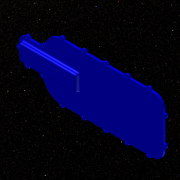
# Autodesk Inventor part: oilcaselid
Saved by Autodesk Inventor 2012 (Build 160160000, 160)
## iProperties
Created: 2012-11-14
Part Number: oilcaselid
Material: Default
Document SubType Name: Modeling
Designer: SONY
Density: 1 g/cm^3
Author: SONY
Autodesk Inventor part; units mm, degrees
ref_plane "YZ Plane" through (0, 0, 0) normal (1, 0, 0) x (0, 1, 0)
ref_plane "XZ Plane" through (0, 0, 0) normal (0, 1, 0) x (-1, 0, 0)
sketch "Sketch1" plane through (0, 0, 0) normal (0, 0, 1) x (1, 0, 0)
  circle A0 centre (150.6134, -24.6977) radius 1.778 projected
  circle A1 centre (150.6134, 24.5422) radius 1.778 projected
  circle A2 centre (122.2034, -53.1077) radius 1.778 projected
  circle A3 centre (122.2034, 52.9522) radius 1.778 projected
  circle A4 centre (-75.7202, -23.3991) radius 1.778 projected
  circle A5 centre (-104.8908, -21.7252) radius 1.778 projected
  circle A6 centre (0.2834, -53.1077) radius 1.778 projected
  circle A7 centre (-40.3566, -53.1077) radius 1.778 projected
  circle A8 centre (81.5634, -53.1077) radius 1.778 projected
  circle A9 centre (40.9234, -53.1077) radius 1.778 projected
  circle A10 centre (81.5634, 52.9522) radius 1.778 projected
  circle A11 centre (40.9234, 52.9522) radius 1.778 projected
  circle A12 centre (0.2834, 52.9522) radius 1.778 projected
  circle A13 centre (-40.3566, 52.9522) radius 1.778 projected
  circle A14 centre (-74.4108, 24.5186) radius 1.778 projected
  circle A15 centre (-104.8908, 22.8448) radius 1.778 projected
  circle A16 centre (-119.9566, 0.5598) radius 1.778 projected
  arc A17 (130.9284, -53.1077) -> (150.6134, -33.4227) centre (130.9284, -33.4227) ccw projected
  line L0 (150.6134, -29.4602) -> (150.6134, -33.4227) projected
  arc A18 (150.6134, -29.4602) -> (150.6134, -19.9352) centre (150.6134, -24.6977) ccw projected
  line L1 (150.6134, 19.7797) -> (150.6134, -19.9352) projected
  arc A19 (150.6134, 19.7797) -> (150.6134, 29.3047) centre (150.6134, 24.5422) ccw projected
  line L2 (150.6134, 33.2672) -> (150.6134, 29.3047) projected
  arc A20 (150.6134, 33.2672) -> (130.9284, 52.9522) centre (130.9284, 33.2672) ccw projected
  line L3 (130.9284, 52.9522) -> (126.9659, 52.9522) projected
  arc A21 (126.9659, 52.9522) -> (117.4409, 52.9522) centre (122.2034, 52.9522) ccw projected
  line L4 (117.4409, 52.9522) -> (86.3259, 52.9522) projected
  arc A22 (86.3259, 52.9522) -> (76.8009, 52.9522) centre (81.5634, 52.9522) ccw projected
  line L5 (76.8009, 52.9522) -> (45.6859, 52.9522) projected
  arc A23 (45.6859, 52.9522) -> (36.1609, 52.9522) centre (40.9234, 52.9522) ccw projected
  line L6 (36.1609, 52.9522) -> (5.0459, 52.9522) projected
  arc A24 (5.0459, 52.9522) -> (-4.4791, 52.9522) centre (0.2834, 52.9522) ccw projected
  line L7 (-4.4791, 52.9522) -> (-35.5941, 52.9522) projected
  arc A25 (-35.5941, 52.9522) -> (-45.107, 52.6131) centre (-40.3566, 52.9522) ccw projected
  arc A26 (-45.107, 52.6131) -> (-72.4622, 28.8643) centre (-40.3566, 19.5123) ccw projected
  arc A27 (-72.4622, 28.8643) -> (-78.8694, 22.8448) centre (-74.4108, 24.5186) ccw projected
  line L8 (-78.8694, 22.8448) -> (-100.1283, 22.8448) projected
  arc A28 (-100.1283, 22.8448) -> (-109.6533, 22.8236) centre (-104.8908, 22.8448) ccw projected
  arc A29 (-109.6533, 22.8236) -> (-119.9566, 11.8598) centre (-108.9716, 11.8598) ccw projected
  line L9 (-119.9566, 11.8598) -> (-119.9566, 5.3223) projected
  arc A30 (-119.9566, 5.3223) -> (-119.9566, -4.2027) centre (-119.9566, 0.5598) ccw projected
  line L10 (-119.9566, -4.2027) -> (-119.9566, -10.7402) projected
  arc A31 (-119.9566, -10.7402) -> (-109.6533, -21.7041) centre (-108.9716, -10.7402) ccw projected
  arc A32 (-109.6533, -21.7041) -> (-100.1283, -21.7252) centre (-104.8908, -21.7252) ccw projected
  line L11 (-100.1283, -21.7252) -> (-80.1788, -21.7252) projected
  arc A33 (-80.1788, -21.7252) -> (-73.7864, -27.7513) centre (-75.7202, -23.3991) ccw projected
  arc A34 (-73.7864, -27.7513) -> (-45.1079, -52.7811) centre (-40.3566, -18.3927) ccw projected
  arc A35 (-45.1079, -52.7811) -> (-35.5941, -53.1077) centre (-40.3566, -53.1077) ccw projected
  line L12 (-35.5941, -53.1077) -> (-4.4791, -53.1077) projected
  arc A36 (-4.4791, -53.1077) -> (5.0459, -53.1077) centre (0.2834, -53.1077) ccw projected
  line L13 (5.0459, -53.1077) -> (36.1609, -53.1077) projected
  arc A37 (36.1609, -53.1077) -> (45.6859, -53.1077) centre (40.9234, -53.1077) ccw projected
  line L14 (45.6859, -53.1077) -> (76.8009, -53.1077) projected
  arc A38 (76.8009, -53.1077) -> (86.3259, -53.1077) centre (81.5634, -53.1077) ccw projected
  line L15 (86.3259, -53.1077) -> (117.4409, -53.1077) projected
  arc A39 (117.4409, -53.1077) -> (126.9659, -53.1077) centre (122.2034, -53.1077) ccw projected
  line L16 (126.9659, -53.1077) -> (130.9284, -53.1077) projected
  arc A40 (-69.8901, -25.1738) -> (-79.7613, -17.3122) centre (-79.7613, -27.4402) ccw projected
  line L17 (-79.7613, -17.3122) -> (-108.9716, -17.3122) projected
  arc A41 (-115.5436, -10.7402) -> (-108.9716, -17.3122) centre (-108.9716, -10.7402) ccw projected
  line L18 (-115.5436, -10.7402) -> (-115.5436, 11.8598) projected
  arc A42 (-108.9716, 18.4318) -> (-115.5436, 11.8598) centre (-108.9716, 11.8598) ccw projected
  line L19 (-108.9716, 18.4318) -> (-78.4519, 18.4318) projected
  arc A43 (-78.4519, 18.4318) -> (-68.598, 26.2195) centre (-78.4519, 28.5598) ccw projected
  arc A44 (-40.3566, 48.5392) -> (-68.598, 26.2195) centre (-40.3566, 19.5123) ccw projected
  line L20 (-40.3566, 48.5392) -> (130.9284, 48.5392) projected
  arc A45 (146.2004, 33.2672) -> (130.9284, 48.5392) centre (130.9284, 33.2672) ccw projected
  line L21 (146.2004, 33.2672) -> (146.2004, -33.4227) projected
  arc A46 (130.9284, -48.6947) -> (146.2004, -33.4227) centre (130.9284, -33.4227) ccw projected
  line L22 (130.9284, -48.6947) -> (-40.3566, -48.6947) projected
  arc A47 (-69.8901, -25.1738) -> (-40.3566, -48.6947) centre (-40.3566, -18.3927) ccw projected
  arc A48 (-108.9716, 15.8918) -> (-113.0036, 11.8598) centre (-108.9716, 11.8598) ccw projected
  line L23 (-113.0036, 11.8598) -> (-113.0036, -10.7402) projected
  arc A49 (-113.0036, -10.7402) -> (-108.9716, -14.7722) centre (-108.9716, -10.7402) ccw projected
  line L24 (-108.9716, -14.7722) -> (-79.7613, -14.7722) projected
  arc A50 (-67.4146, -24.6054) -> (-79.7613, -14.7722) centre (-79.7613, -27.4402) ccw projected
  arc A51 (-67.4146, -24.6054) -> (-40.3566, -46.1547) centre (-40.3566, -18.3927) ccw projected
  line L25 (-40.3566, -46.1547) -> (130.9284, -46.1547) projected
  arc A52 (130.9284, -46.1547) -> (143.6604, -33.4227) centre (130.9284, -33.4227) ccw projected
  line L26 (143.6604, -33.4227) -> (143.6604, 33.2672) projected
  arc A53 (143.6604, 33.2672) -> (130.9284, 45.9992) centre (130.9284, 33.2672) ccw projected
  line L27 (130.9284, 45.9992) -> (-40.3566, 45.9992) projected
  arc A54 (-40.3566, 45.9992) -> (-66.1267, 25.6326) centre (-40.3566, 19.5123) ccw projected
  arc A55 (-78.4519, 15.8918) -> (-66.1267, 25.6326) centre (-78.4519, 28.5598) ccw projected
  line L28 (-78.4519, 15.8918) -> (-108.9716, 15.8918) projected
  arc A56 (130.9284, -44.1227) -> (141.6284, -33.4227) centre (130.9284, -33.4227) ccw projected
  line L29 (97.7484, -44.1227) -> (130.9284, -44.1227) projected
  arc A57 (95.8628, -42.7894) -> (97.7484, -44.1227) centre (97.7484, -42.1227) ccw projected
  arc A58 (95.8628, -42.7894) -> (94.92, -42.1227) centre (94.92, -43.1227) ccw projected
  line L30 (94.92, -42.1227) -> (94.7484, -42.1227) projected
  arc A59 (94.7484, -42.1227) -> (93.7484, -43.1227) centre (94.7484, -43.1227) ccw projected
  line L31 (93.7484, -44.1227) -> (93.7484, -43.1227) projected
  line L32 (90.5734, -44.1227) -> (93.7484, -44.1227) projected
  line L33 (90.5734, -44.1227) -> (90.5734, -43.1227) projected
  arc A60 (90.5734, -43.1227) -> (89.5734, -42.1227) centre (89.5734, -43.1227) ccw projected
  line L34 (89.5734, -42.1227) -> (83.9534, -42.1227) projected
  arc A61 (83.9534, -42.1227) -> (82.9534, -43.1227) centre (83.9534, -43.1227) ccw projected
  line L35 (82.9534, -44.1227) -> (82.9534, -43.1227) projected
  line L36 (79.7784, -44.1227) -> (82.9534, -44.1227) projected
  line L37 (79.7784, -44.1227) -> (79.7784, -43.1227) projected
  arc A62 (79.7784, -43.1227) -> (78.7784, -42.1227) centre (78.7784, -43.1227) ccw projected
  line L38 (78.7784, -42.1227) -> (73.1584, -42.1227) projected
  arc A63 (73.1584, -42.1227) -> (72.1584, -43.1227) centre (73.1584, -43.1227) ccw projected
  line L39 (72.1584, -44.1227) -> (72.1584, -43.1227) projected
  line L40 (68.9834, -44.1227) -> (72.1584, -44.1227) projected
  line L41 (68.9834, -44.1227) -> (68.9834, -43.1227) projected
  arc A64 (68.9834, -43.1227) -> (67.9834, -42.1227) centre (67.9834, -43.1227) ccw projected
  line L42 (67.9834, -42.1227) -> (67.8118, -42.1227) projected
  arc A65 (67.8118, -42.1227) -> (66.869, -42.7894) centre (67.8118, -43.1227) ccw projected
  arc A66 (64.9834, -44.1227) -> (66.869, -42.7894) centre (64.9834, -42.1227) ccw projected
  line L43 (33.4234, -44.1227) -> (64.9834, -44.1227) projected
  arc A67 (31.5378, -42.7894) -> (33.4234, -44.1227) centre (33.4234, -42.1227) ccw projected
  arc A68 (31.5378, -42.7894) -> (30.595, -42.1227) centre (30.595, -43.1227) ccw projected
  line L44 (30.595, -42.1227) -> (30.4234, -42.1227) projected
  arc A69 (30.4234, -42.1227) -> (29.4234, -43.1227) centre (30.4234, -43.1227) ccw projected
  line L45 (29.4234, -44.1227) -> (29.4234, -43.1227) projected
  line L46 (26.2484, -44.1227) -> (29.4234, -44.1227) projected
  line L47 (26.2484, -44.1227) -> (26.2484, -43.1227) projected
  arc A70 (26.2484, -43.1227) -> (25.2484, -42.1227) centre (25.2484, -43.1227) ccw projected
  line L48 (25.2484, -42.1227) -> (25.0768, -42.1227) projected
  arc A71 (25.0768, -42.1227) -> (24.134, -42.7894) centre (25.0768, -43.1227) ccw projected
  arc A72 (22.2484, -44.1227) -> (24.134, -42.7894) centre (22.2484, -42.1227) ccw projected
  line L49 (-40.3566, -44.1227) -> (22.2484, -44.1227) projected
  arc A73 (-65.4341, -24.1506) -> (-40.3566, -44.1227) centre (-40.3566, -18.3927) ccw projected
  arc A74 (-65.4341, -24.1506) -> (-79.7613, -12.7402) centre (-79.7613, -27.4402) ccw projected
  line L50 (-108.9716, -12.7402) -> (-79.7613, -12.7402) projected
  arc A75 (-110.9716, -10.7402) -> (-108.9716, -12.7402) centre (-108.9716, -10.7402) ccw projected
  line L51 (-110.9716, 11.8598) -> (-110.9716, -10.7402) projected
  arc A76 (-108.9716, 13.8598) -> (-110.9716, 11.8598) centre (-108.9716, 11.8598) ccw projected
  line L52 (-78.4519, 13.8598) -> (-108.9716, 13.8598) projected
  arc A77 (-78.4519, 13.8598) -> (-64.1497, 25.163) centre (-78.4519, 28.5598) ccw projected
  arc A78 (-40.3566, 43.9672) -> (-64.1497, 25.163) centre (-40.3566, 19.5123) ccw projected
  line L53 (22.2484, 43.9672) -> (-40.3566, 43.9672) projected
  arc A79 (24.134, 42.6339) -> (22.2484, 43.9672) centre (22.2484, 41.9672) ccw projected
  arc A80 (24.134, 42.6339) -> (25.0768, 41.9672) centre (25.0768, 42.9672) ccw projected
  line L54 (25.0768, 41.9672) -> (25.2484, 41.9672) projected
  arc A81 (25.2484, 41.9672) -> (26.2484, 42.9672) centre (25.2484, 42.9672) ccw projected
  line L55 (26.2484, 43.9672) -> (26.2484, 42.9672) projected
  line L56 (29.4234, 43.9672) -> (26.2484, 43.9672) projected
  line L57 (29.4234, 43.9672) -> (29.4234, 42.9672) projected
  arc A82 (29.4234, 42.9672) -> (30.4234, 41.9672) centre (30.4234, 42.9672) ccw projected
  line L58 (30.4234, 41.9672) -> (30.595, 41.9672) projected
  arc A83 (30.595, 41.9672) -> (31.5378, 42.6339) centre (30.595, 42.9672) ccw projected
  arc A84 (33.4234, 43.9672) -> (31.5378, 42.6339) centre (33.4234, 41.9672) ccw projected
  line L59 (64.9834, 43.9672) -> (33.4234, 43.9672) projected
  arc A85 (66.869, 42.6339) -> (64.9834, 43.9672) centre (64.9834, 41.9672) ccw projected
  arc A86 (66.869, 42.6339) -> (67.8118, 41.9672) centre (67.8118, 42.9672) ccw projected
  line L60 (67.8118, 41.9672) -> (67.9834, 41.9672) projected
  arc A87 (67.9834, 41.9672) -> (68.9834, 42.9672) centre (67.9834, 42.9672) ccw projected
  line L61 (68.9834, 43.9672) -> (68.9834, 42.9672) projected
  line L62 (72.1584, 43.9672) -> (68.9834, 43.9672) projected
  line L63 (72.1584, 43.9672) -> (72.1584, 42.9672) projected
  arc A88 (72.1584, 42.9672) -> (73.1584, 41.9672) centre (73.1584, 42.9672) ccw projected
  line L64 (73.1584, 41.9672) -> (78.7784, 41.9672) projected
  arc A89 (78.7784, 41.9672) -> (79.7784, 42.9672) centre (78.7784, 42.9672) ccw projected
  line L65 (79.7784, 43.9672) -> (79.7784, 42.9672) projected
  line L66 (82.9534, 43.9672) -> (79.7784, 43.9672) projected
  line L67 (82.9534, 43.9672) -> (82.9534, 42.9672) projected
  arc A90 (82.9534, 42.9672) -> (83.9534, 41.9672) centre (83.9534, 42.9672) ccw projected
  line L68 (83.9534, 41.9672) -> (89.5734, 41.9672) projected
  arc A91 (89.5734, 41.9672) -> (90.5734, 42.9672) centre (89.5734, 42.9672) ccw projected
  line L69 (90.5734, 43.9672) -> (90.5734, 42.9672) projected
  line L70 (93.7484, 43.9672) -> (90.5734, 43.9672) projected
  line L71 (93.7484, 43.9672) -> (93.7484, 42.9672) projected
  arc A92 (93.7484, 42.9672) -> (94.7484, 41.9672) centre (94.7484, 42.9672) ccw projected
  line L72 (94.7484, 41.9672) -> (94.92, 41.9672) projected
  arc A93 (94.92, 41.9672) -> (95.8628, 42.6339) centre (94.92, 42.9672) ccw projected
  arc A94 (97.7484, 43.9672) -> (95.8628, 42.6339) centre (97.7484, 41.9672) ccw projected
  line L73 (130.9284, 43.9672) -> (97.7484, 43.9672) projected
  arc A95 (141.6284, 33.2672) -> (130.9284, 43.9672) centre (130.9284, 33.2672) ccw projected
  line L74 (141.6284, 33.2672) -> (141.6284, -33.4227) projected
  arc A96 (-108.9716, 15.8918) -> (-113.0036, 11.8598) centre (-108.9716, 11.8598) ccw projected
  line L75 (-78.4519, 15.8918) -> (-108.9716, 15.8918) projected
  arc A97 (-78.4519, 15.8918) -> (-66.1267, 25.6326) centre (-78.4519, 28.5598) ccw projected
  arc A98 (-40.3566, 45.9992) -> (-66.1267, 25.6326) centre (-40.3566, 19.5123) ccw projected
  line L76 (130.9284, 45.9992) -> (-40.3566, 45.9992) projected
  arc A99 (143.6604, 33.2672) -> (130.9284, 45.9992) centre (130.9284, 33.2672) ccw projected
  line L77 (143.6604, -33.4227) -> (143.6604, 33.2672) projected
  arc A100 (130.9284, -46.1547) -> (143.6604, -33.4227) centre (130.9284, -33.4227) ccw projected
  line L78 (-40.3566, -46.1547) -> (130.9284, -46.1547) projected
  arc A101 (-67.4146, -24.6054) -> (-40.3566, -46.1547) centre (-40.3566, -18.3927) ccw projected
  arc A102 (-67.4146, -24.6054) -> (-79.7613, -14.7722) centre (-79.7613, -27.4402) ccw projected
  line L79 (-108.9716, -14.7722) -> (-79.7613, -14.7722) projected
  arc A103 (-113.0036, -10.7402) -> (-108.9716, -14.7722) centre (-108.9716, -10.7402) ccw projected
  line L80 (-113.0036, 11.8598) -> (-113.0036, -10.7402) projected
  arc A104 (-69.8901, -25.1738) -> (-79.7613, -17.3122) centre (-79.7613, -27.4402) ccw projected
  arc A105 (-69.8901, -25.1738) -> (-40.3566, -48.6947) centre (-40.3566, -18.3927) ccw projected
  line L81 (-40.3566, -48.6947) -> (130.9284, -48.6947) projected
  arc A106 (130.9284, -48.6947) -> (146.2004, -33.4227) centre (130.9284, -33.4227) ccw projected
  line L82 (146.2004, -33.4227) -> (146.2004, 33.2672) projected
  arc A107 (146.2004, 33.2672) -> (130.9284, 48.5392) centre (130.9284, 33.2672) ccw projected
  line L83 (130.9284, 48.5392) -> (-40.3566, 48.5392) projected
  arc A108 (-40.3566, 48.5392) -> (-68.598, 26.2195) centre (-40.3566, 19.5123) ccw projected
  arc A109 (-78.4519, 18.4318) -> (-68.598, 26.2195) centre (-78.4519, 28.5598) ccw projected
  line L84 (-78.4519, 18.4318) -> (-108.9716, 18.4318) projected
  arc A110 (-108.9716, 18.4318) -> (-115.5436, 11.8598) centre (-108.9716, 11.8598) ccw projected
  line L85 (-115.5436, 11.8598) -> (-115.5436, -10.7402) projected
  arc A111 (-115.5436, -10.7402) -> (-108.9716, -17.3122) centre (-108.9716, -10.7402) ccw projected
  line L86 (-108.9716, -17.3122) -> (-79.7613, -17.3122) projected
  line L87 (94.7484, -42.1227) -> (67.8118, -42.1227)
  line L88 (30.595, -42.1227) -> (25.2484, -42.1227)
  line L89 (67.9834, 41.9672) -> (94.92, 41.9672)
  line L90 (30.4234, 41.9672) -> (25.0768, 41.9672)
  constraints: 12 tangent, 8 end point, 2 collinear, 2 parallel, 2 point on circle, 42 other
extrude "Extrusion1" add sketch "Sketch1" along normal blind 4 contours L16 A39 L15 A38 L14 A37 L13 A36 L12 A35 A34 A33 L11 A32 A31 L10 A30 L9 A29 A28 L8 A27 A26 A25 L7 A24 L6 A23 L5 A22 L4 A21 L3 A20 L2 A19 L1 A18 L0 A17 | A40 L17 A41 L18 A42 L19 A43 A44 L20 A45 L21 A46 L22 A47 | L28 A55 A54 L27 A53 L26 A52 L25 A51 A50 L24 A49 L23 A48 | L29 A57 A58 L30 L87 L34 L38 L42 A65 A66 L43 A67 A68 L44 L88 L48 A71 A72 L49 A73 A74 L50 A75 L51 A76 L52 A77 A78 L53 A79 A80 L54 L90 L58 A83 A84 L59 A85 A86 L60 L89 L64 L68 L72 A93 A94 L73 A95 L74 A56 | A59 L31 L32 L33 A60 L87 | A61 L35 L36 L37 A62 L87 | L89 A91 L69 L70 L71 A92 | A63 L39 L40 L41 A64 L87 | L89 A89 L65 L66 L67 A90 | L89 A87 L61 L62 L63 A88 | A69 L45 L46 L47 A70 L88 | L90 A81 L55 L56 L57 A82
fillet "Fillet7" radius 3.175 34 edges at (150.6134, 19.7797, 2) (150.6134, 29.3047, 2) (150.6134, -19.9352, 2) (150.6134, -29.4602, 2) (126.9659, -53.1077, 2) (117.4409, -53.1077, 2) (86.3259, -53.1077, 2) (76.8009, -53.1077, 2) (5.0459, -53.1077, 2) (45.6859, -53.1077, 2) (36.1609, -53.1077, 2) (-4.4791, -53.1077, 2) (-35.5941, -53.1077, 2) (-45.1079, -52.7811, 2) (-73.7864, -27.7513, 2) (-80.1788, -21.7252, 2) (-100.1283, -21.7252, 2) (-109.6533, -21.7041, 2) (-119.9566, -4.2027, 2) (-119.9566, 5.3223, 2) (-78.8694, 22.8448, 2) (-72.4622, 28.8643, 2) (-100.1283, 22.8448, 2) (-109.6533, 22.8236, 2) (-4.4791, 52.9522, 2) (5.0459, 52.9522, 2) (-35.5941, 52.9522, 2) (-45.107, 52.6131, 2) (45.6859, 52.9522, 2) (36.1609, 52.9522, 2) (76.8009, 52.9522, 2) (86.3259, 52.9522, 2) (117.4409, 52.9522, 2) (126.9659, 52.9522, 2)
sketch "Sketch9" plane through (0, 0, 4) normal (0, 0, 1) x (1, 0, 0)
  arc A0 (-110.9716, -10.7402) -> (-108.9716, -12.7402) centre (-108.9716, -10.7402) ccw projected
  line L0 (-108.9716, -12.7402) -> (-8.1716, -12.7402) projected
  line L1 (-8.1716, -12.7402) -> (-8.1716, 13.8598) projected
  line L2 (-8.1716, 13.8598) -> (-108.9716, 13.8598) projected
  arc A1 (-108.9716, 13.8598) -> (-110.9716, 11.8598) centre (-108.9716, 11.8598) ccw projected
  line L3 (-110.9716, -10.7402) -> (-110.9716, 11.8598) projected
  point P0 (0, 0)
extrude "Extrusion9" cut sketch "Sketch9" against normal through all
sketch "Sketch10" plane through (0, 0, 4) normal (0, 0, 1) x (1, 0, 0)
  arc A0 (130.9284, -53.1077) -> (150.6134, -33.4227) centre (130.9284, -33.4227) ccw projected
  arc A1 (-40.3566, 43.9672) -> (-64.1497, 25.163) centre (-40.3566, 19.5123) ccw projected
  line L0 (22.2484, 43.9672) -> (-40.3566, 43.9672) projected
  arc A2 (-78.4519, 13.8598) -> (-64.1497, 25.163) centre (-78.4519, 28.5598) ccw projected
  line L1 (-40.3566, -44.1227) -> (22.2484, -44.1227) projected
  line L2 (33.4234, -44.1227) -> (67.5159, -44.1227) projected
  line L3 (67.5159, 43.9672) -> (33.4234, 43.9672) projected
  arc A3 (-65.4341, -24.1506) -> (-79.7613, -12.7402) centre (-79.7613, -27.4402) ccw projected
  line L4 (130.9284, 43.9672) -> (96.9309, 43.9672) projected
  line L5 (141.6284, 33.2672) -> (141.6284, -33.4227) projected
  arc A4 (130.9284, -44.1227) -> (141.6284, -33.4227) centre (130.9284, -33.4227) ccw projected
  line L6 (96.9309, -44.1227) -> (130.9284, -44.1227) projected
  arc A5 (141.6284, 33.2672) -> (130.9284, 43.9672) centre (130.9284, 33.2672) ccw projected
  line L7 (96.9309, -44.1227) -> (67.5159, -44.1227)
  line L8 (33.4234, -44.1227) -> (22.2484, -44.1227)
  line L9 (22.2484, 43.9672) -> (33.4234, 43.9672)
  line L10 (67.5159, 43.9672) -> (96.9309, 43.9672)
  line L11 (130.9284, 33.2672) -> (54.7284, 33.2672)
  line L12 (54.7284, 33.2672) -> (54.7284, -33.4227)
  line L13 (54.7284, -33.4227) -> (130.9284, -33.4227)
  line L14 (130.9284, -33.4227) -> (130.9284, 33.2672)
  arc A6 (-65.4341, -24.1506) -> (-40.3566, -44.1227) centre (-40.3566, -18.3927) ccw projected
  point P0 (0, 0)
  dimension "d32" = 76.2
  constraints: 16 end point, 3 collinear, 3 parallel, 1 coincident, 1 horizontal, 1 perpendicular
  measures "d32" distance of L12.end L13.end
extrude "Extrusion10" cut sketch "Sketch10" against normal through all
fillet "Fillet8" radius 6.35 4 edges at (54.7284, 33.2672, 2) (130.9284, -33.4227, 2) (54.7284, -33.4227, 2) (130.9284, 33.2672, 2)
sketch "Sketch11" plane through (0, 0, 4) normal (0, 0, 1) x (1, 0, 0)
  line L0 (-8.1716, -12.7402) -> (-108.9716, -12.7402) projected
  arc A0 (-110.9716, -10.7402) -> (-108.9716, -12.7402) centre (-108.9716, -10.7402) ccw projected
  line L1 (-110.9716, -10.7402) -> (-110.9716, 11.8598) projected
  arc A1 (-108.9716, 13.8598) -> (-110.9716, 11.8598) centre (-108.9716, 11.8598) ccw projected
  line L2 (-108.9716, 13.8598) -> (-8.1716, 13.8598) projected
  line L3 (-8.1716, 13.8598) -> (-8.1716, -12.7402) projected
  line L4 (-112.9716, 15.8598) -> (-6.1716, 15.8598)
  line L5 (-6.1716, 15.8598) -> (-6.1716, -14.7402)
  line L6 (-6.1716, -14.7402) -> (-112.9716, -14.7402)
  line L7 (-112.9716, -14.7402) -> (-112.9716, 15.8598)
  line L8 (-107.1966, -12.1402) -> (-11.9466, -12.1402) projected
  line L9 (-11.9466, 13.2598) -> (-11.9466, -12.1402) projected
  line L10 (-107.1966, 13.2598) -> (-11.9466, 13.2598) projected
  line L11 (-107.1966, 13.2598) -> (-107.1966, -12.1402) projected
  point P0 (0, 0)
  dimension "d36" = 2
  dimension "d37" = 2
  dimension "d38" = 2
  dimension "d39" = 2
  dimension "d40" = 0.6
  constraints: 8 end point, 2 parallel, 1 horizontal, 1 perpendicular
  measures "d36" distance between parallel lines of L0 L6
  measures "d37" distance between parallel lines of L2 L4
  measures "d38" distance between parallel lines of L5 L3
  measures "d39" distance between parallel lines of L7 L1
  measures "d40" distance between parallel lines of L2 L10
ref_plane "Work Plane2" through (-107.1966, 13.2598, 10.7696) normal (0, 0, 1) x (-1, 0, 0)
ref_plane "Work Plane3" through (-107.1966, 13.2598, 11.3538) normal (0, 0, 1) x (-1, 0, 0)
extrude "Extrusion11" add sketch "Sketch11" along normal up to surface (7.3538 mm away) contours L4 L5 L6 L7
sketch "Sketch12" plane through (-112.9716, 15.8598, 11.3538) normal (0, 0, 1) x (1, 0, 0)
  line L0 (106.8, 0) -> (106.8, -30.6) projected
  line L1 (0, 0) -> (106.8, 0) projected
  line L2 (0, -30.6) -> (0, 0) projected
  line L3 (106.8, -30.6) -> (0, -30.6) projected
  point P0 (112.9716, -15.8598)
extrude "Extrusion12" add sketch "Sketch12" along normal blind 2
fillet "Fillet9" radius 2 12 edges at (-112.9716, 15.8598, 8.6769) (-112.9716, -14.7402, 8.6769) (-6.1716, 15.8598, 8.6769) (-6.1716, -14.7402, 8.6769) (-112.9716, 0.5598, 4) (-59.5716, 15.8598, 4) (-6.1716, 0.5598, 4) (-59.5716, -14.7402, 4) (-59.5716, -14.7402, 13.3538) (-6.1716, 0.5598, 13.3538) (-59.5716, 15.8598, 13.3538) (-112.9716, 0.5598, 13.3538)
equation "\"d1\" = 2 * thickness"
equation "\"thickness\" = 2"
body "Solid1"
